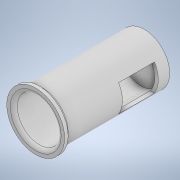
# Autodesk Inventor part: Peça1
Saved by Autodesk Inventor 2022 (Build 260153000, 153)
## iProperties
Created: 2023-10-22
Part Number: Peça1
Material: Genérico
Document SubType Name: Modeling
Designer: Daniel
Density: 1 g/cm^3
Appearance: Padrão
Author: Daniel
Autodesk Inventor part; units mm, degrees
ref_plane "XZ Plane" through (0, 0, 0) normal (0, 1, 0) x (-1, 0, 0)
ref_plane "XY Plane" through (0, 0, 0) normal (0, 0, 1) x (1, 0, 0)
sketch "Esboço1" plane through (0, 0, 0) normal (0, 0, 1) x (1, 0, 0)
  circle A0 centre (0, 0) radius 14.5
  dimension "d0" = 29
  constraints: 1 centre point, 1 coincident
  measures "d0" diameter of A0
extrude "Extrusão1" add sketch "Esboço1" along normal blind 2
sketch "Esboço2" plane through (0, 0, 2) normal (0, 0, 1) x (1, 0, 0)
  circle A0 centre (0, 0) radius 14.5 projected
  circle A1 centre (0, 0) radius 12.5
  dimension "d3" = 2
  constraints: 1 centre point
  measures "d3" radial gap between concentric circles of A0 A1
extrude "Extrusão2" add sketch "Esboço2" along normal blind 58
ref_plane "Plano de trabalho4" through (29, 0, 0) normal (1, 0, 0) x (0, 1, 0)
sketch "Esboço5" plane through (29, 0, 0) normal (1, 0, 0) x (0, 1, 0)
  line L0 (-7.75, 27) -> (7.75, 27)
  line L1 (7.75, 27) -> (7.75, 6.5)
  line L2 (7.75, 6.5) -> (-7.75, 6.5)
  line L3 (-7.75, 6.5) -> (-7.75, 27)
  line L4 (-7.75, 27) -> (7.75, 6.5) construction
  line L5 (7.75, 27) -> (-7.75, 6.5) construction
  line L6 (14.5, 0) -> (-14.5, 0) projected
  point P0 (0, 0)
  point P1 (0, 16.75)
  dimension "d15" = 20.5
  dimension "d16" = 15.5
  dimension "d17" = 0
  dimension "d18" = 6.5
  constraints: 12 end point, 2 midpoint, 2 parallel, 1 horizontal, 1 perpendicular
  measures "d15" distance of L0.end L1.end
  measures "d16" distance of L1.end L2.end
  measures "d17" horizontal distance of point (0, 0) point (0, 16.75)
  measures "d18" distance between parallel lines of L6 L2
extrude "Extrusão4" cut sketch "Esboço5" against normal through all
sketch "Esboço7" plane through (0, 0, 60) normal (0, 0, 1) x (1, 0, 0)
  circle A0 centre (0, 0) radius 16.5
  circle A1 centre (0, 0) radius 12.5 projected
  dimension "d28" = 33
  constraints: 1 centre point, 1 coincident
  measures "d28" diameter of A0
extrude "Extrusão6" add sketch "Esboço7" along normal blind 2
fillet "Arredondamento2" radius 2 1 edges at (-12.5, 0, 62)
fillet "Arredondamento3" radius 2 1 edges at (-14.5, 0, 60)
